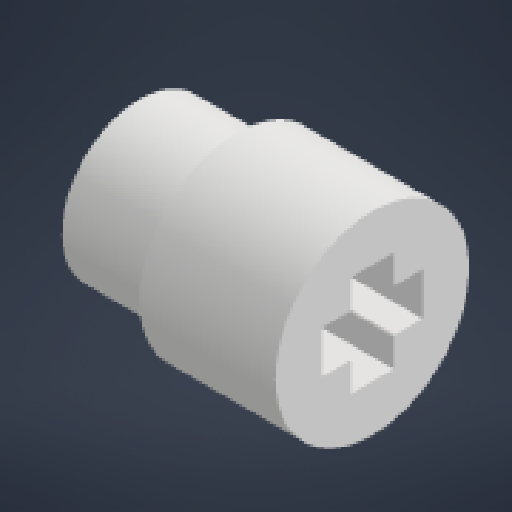
# Autodesk Inventor part: AcopleMotor
Saved by Autodesk Inventor 2026.3 (Build 303398000, 398)
## iProperties
Created: 2026-04-28
Part Number: AcopleMotor
Material: Genérico
Document SubType Name: Modeling
Designer: Jose Carlos
Density: 1 g/cm^3
Appearance: Valor por defecto
Author: Jose Carlos
Autodesk Inventor part; units mm, degrees
ref_plane "YZ Plane" through (0, 0, 0) normal (1, 0, 0) x (0, 1, 0)
ref_plane "XZ Plane" through (0, 0, 0) normal (0, 1, 0) x (-1, 0, 0)
ref_plane "XY Plane" through (0, 0, 0) normal (0, 0, 1) x (1, 0, 0)
sketch "Boceto1" plane through (0, 0, 0) normal (1, 0, 0) x (0, 1, 0)
  circle A0 centre (0, 0) radius 2.9
  line L0 (0, 5) -> (0, 5)
  line L1 (5, 0) -> (5, 0)
  line L2 (0, -5) -> (0, -5)
  line L3 (-5, 0) -> (-5, 0)
  circle A1 centre (0, 0) radius 4
  dimension "d0" = 5.8
  dimension "d11" = 8
  constraints: 8 end point, 2 centre point, 2 coincident, 2 parallel, 1 horizontal, 1 perpendicular
  measures "d0" diameter of A0
  measures "d11" diameter of A1
extrude "Extrusión1" add sketch "Boceto1" along normal blind 5
sketch "Boceto2" plane through (5, 0, 0) normal (1, 0, 0) x (0, 0, -1)
  line L0 (1.1, -2.6) -> (-1.1, -2.6)
  line L1 (-1.1, -2.6) -> (-1.1, 2.6)
  line L2 (-1.1, 2.6) -> (1.1, 2.6)
  line L3 (1.1, 2.6) -> (1.1, -2.6)
  line L4 (1.1, -2.6) -> (-1.1, 2.6)
  line L5 (-1.1, -2.6) -> (1.1, 2.6)
  line L6 (2.6, -1.1) -> (-2.6, -1.1)
  line L7 (-2.6, -1.1) -> (-2.6, 1.1)
  line L8 (-2.6, 1.1) -> (2.6, 1.1)
  line L9 (2.6, 1.1) -> (2.6, -1.1)
  line L10 (2.6, -1.1) -> (-2.6, 1.1)
  line L11 (-2.6, -1.1) -> (2.6, 1.1)
  circle A0 centre (0, 0) radius 1.6
  circle A1 centre (0, 0) radius 4 projected
  circle A2 centre (0, 0) radius 4
  point P0 (-1.1, -1.1619)
  point P1 (-1.1619, -1.1)
  point P2 (-1.1619, 1.1)
  point P3 (-1.1, 1.1619)
  point P4 (1.1, 1.1619)
  point P5 (1.1619, 1.1)
  point P6 (1.1619, -1.1)
  point P7 (1.1, -1.1619)
  dimension "d6" = 2.2
  dimension "d7" = 5.2
  dimension "d8" = 3.2
  constraints: 24 end point, 4 midpoint, 4 parallel, 4 perpendicular, 2 centre point, 2 coincident, 2 horizontal, 1 concentric
  measures "d6" distance of L1.end L2.end
  measures "d7" distance of L0.end L1.end
  measures "d8" diameter of A0
extrude "Extrusión2" add sketch "Boceto2" along normal blind 7
